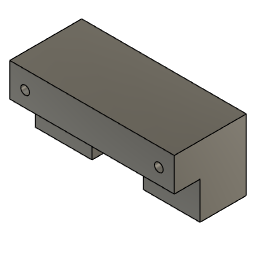
water leakage point stand (Autodesk Fusion 360 design; units mm, degrees)
Autodesk Fusion 360 part; units mm, degrees
sketch "Sketch1" plane through (0, 0, 0) normal (0, 0, 1) x (1, 0, 0)
  line L0 (0, 0) -> (64, 0)
  line L1 (64, 0) -> (64, 28)
  line L2 (64, 28) -> (0, 28)
  line L3 (0, 28) -> (0, 0)
  line L4 (0, 0) -> (0, 10)
  line L5 (0, 10) -> (64, 10)
  line L6 (32, 28) -> (42, 28)
  line L7 (32, 28) -> (22, 28)
  line L8 (22, 28) -> (42, 28)
  line L9 (42, 28) -> (42, 10)
  line L10 (42, 10) -> (22, 10)
  line L11 (22, 10) -> (22, 28)
  point P0 (32, 28)
  dimension "d1" = 64
  dimension "d2" = 28
  dimension "d3" = 10
  constraint horizontal L0
  constraint vertical L1
  constraint horizontal L2
  constraint vertical L3
  constraint coincident L0.start L3.end
  constraint perpendicular L0 L4
  constraint coincident L1 L5.end
  constraint perpendicular L1 L5
  constraint midpoint L2 P0
  constraint coincident P0 L6.start
  constraint coincident L2 L6.end
  constraint parallel L2 L6
  constraint coincident L2 L7.end
  constraint horizontal L8
  constraint vertical L9
  constraint horizontal L10
  constraint vertical L11
  constraint coincident L5 L9.end
  measures "d1" distance of L0.start L0.end
  measures "d2" distance of L0.start L2.end
  measures "d3" distance of L0.start L4.end
extrude "Extrude1" add sketch "Sketch1" along normal blind 27.5
extrude "Extrude2" cut sketch "Sketch1" along normal blind 14.5 contours L0 L1 L3 L4 L5 L10
sketch "Sketch2" plane through (0, 0, 0) normal (0, -1, 0) x (1, 0, 0)
  line L0 (0, 14.5) -> (64, 14.5)
  line L1 (64, 14.5) -> (64, 27.5)
  line L2 (64, 27.5) -> (0, 27.5)
  line L3 (0, 27.5) -> (0, 14.5)
  line L4 (64, 14.5) -> (58, 14.5) construction
  line L5 (64, 14.5) -> (64, 20.5) construction
  line L6 (0, 14.5) -> (6, 14.5)
  line L7 (0, 14.5) -> (0, 20.5)
  point P0 (58, 20.5)
  point P1 (6, 20.5)
  dimension "d8" = 6
  dimension "d9" = 6
  dimension "d10" = 6
  dimension "d11" = 6
  constraint coincident L0.end L1.start
  constraint perpendicular L1 L4
  constraint perpendicular L4 L5
  constraint coincident L0.start L3.end
  constraint perpendicular L3 L6
  constraint perpendicular L0 L7
  measures "d8" distance of L0.end L4.end
  measures "d9" distance of L0.end L5.end
  measures "d10" distance of L0.start L6.end
  measures "d11" distance of L0.start L7.end
hole "Hole1" at (6, 0, 20.5) direction (0, 1, 0) diameter 3.4 depth 10 tip angle 118
hole "Hole2" at (58, 0, 20.5) direction (0, 1, 0) diameter 3.4 depth 10 tip angle 118
extrude "Extrude3" cut sketch "Sketch1" along normal blind 10 contours L2 L5 L6 L7 L8 L9 L10 L11
named bodies: "stand"
